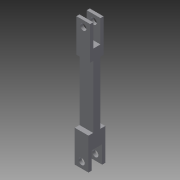
# Autodesk Inventor part: LowerLeg_v2
Saved by Autodesk Inventor 2013 (Build 170138000, 138)
## iProperties
Created: 2012-11-28
Part Number: LowerLeg_v2
Material: Generic
Document SubType Name: Modeling
Designer: Joe
Density: 1 g/cm^3
Author: Joe
Autodesk Inventor part; units mm, degrees
ref_plane "YZ Plane" through (0, 0, 0) normal (1, 0, 0) x (0, 1, 0)
ref_plane "XZ Plane" through (0, 0, 0) normal (0, 1, 0) x (-1, 0, 0)
ref_plane "XY Plane" through (0, 0, 0) normal (0, 0, 1) x (1, 0, 0)
sketch "Sketch1" plane through (0, 0, 0) normal (1, 0, 0) x (0, 1, 0)
  circle A0 centre (0, 0) radius 10
  circle A1 centre (-380, 0) radius 10
  line L0 (0, 0) -> (-380, 0) construction
  line L1 (20, 22.5) -> (-400, 22.5)
  line L2 (-400, 22.5) -> (-400, -22.5)
  line L3 (-400, -22.5) -> (20, -22.5)
  line L4 (20, -22.5) -> (20, 22.5)
  line L5 (20, 0) -> (-400, 0) construction
  dimension "d0" = 380
  dimension "d2" = 20
  dimension "d3" = 20
  dimension "d4" = 20
  dimension "d5" = 20
  dimension "d6" = 45
  constraints: 12 end point, 2 centre point, 2 horizontal, 2 midpoint, 2 parallel, 1 coincident, 1 collinear, 1 perpendicular
  measures "d0" distance of L0.start L0.end
  measures "d2" distance from line of L4 L0.start
  measures "d3" distance from line of L2 L0.end
  measures "d4" diameter of A0
  measures "d5" diameter of A1
  measures "d6" distance of L3.end L1.start
extrude "Extrusion1" add sketch "Sketch1" along normal mid plane 24
sketch "Sketch2" plane through (12, 0, 0) normal (1, 0, 0) x (0, 0, -1)
  circle A0 centre (0, 0) radius 10 projected
  line L0 (22.5, -400) -> (22.5, 20) projected
  line L1 (22.5, 20) -> (-22.5, 20) projected
  line L2 (-22.5, 20) -> (22.5, 20)
  line L3 (22.5, 20) -> (22.5, -90)
  line L4 (22.5, -90) -> (-22.5, -90)
  line L5 (-22.5, -90) -> (-22.5, 20)
  circle A1 centre (0, 0) radius 10
  dimension "d9" = 110
  constraints: 8 end point, 2 parallel, 1 centre point, 1 coincident, 1 concentric, 1 horizontal, 1 perpendicular, 1 point on line
  measures "d9" distance of L4.end L1.end
extrude "Extrusion2" add sketch "Sketch2" along normal blind 10
mirror "Mirror1" about plane through (0, 0, 0) normal (1, 0, 0) of "Extrusion2"
sketch "Sketch3" plane through (-12, -400, 22.5) normal (0, 0, 1) x (1, 0, 0)
  line L0 (34, 420) -> (-10, 420) projected
  line L1 (0, 420) -> (24, 420)
  line L2 (24, 420) -> (24, 345)
  line L3 (24, 345) -> (0, 345)
  line L4 (0, 345) -> (0, 420)
  line L5 (12, 420) -> (12, 345) construction
  point P0 (12, 400)
  dimension "d12" = 24
  dimension "d14" = 75
  constraints: 10 end point, 2 midpoint, 2 parallel, 2 point on line, 1 horizontal, 1 perpendicular
  measures "d12" distance of L2.end L3.end
  measures "d14" distance of L3.end L1.start
extrude "Extrusion3" cut sketch "Sketch3" against normal through all
sketch "Sketch4" plane through (12, 0, 0) normal (1, 0, 0) x (0, 0, -1)
  line L0 (22.5, -400) -> (22.5, -90) projected
  circle A0 centre (0, -380) radius 10 projected
  line L1 (-22.5, -400) -> (22.5, -400)
  line L2 (22.5, -400) -> (22.5, -295)
  line L3 (22.5, -295) -> (-22.5, -295)
  line L4 (-22.5, -295) -> (-22.5, -400)
  circle A1 centre (0, -380) radius 10
  point P0 (0, 0)
  dimension "d18" = 85
  constraints: 8 end point, 2 parallel, 1 centre point, 1 coincident, 1 concentric, 1 horizontal, 1 perpendicular, 1 point on line
  measures "d18" distance from line of A0.centre L3
extrude "Extrusion4" add sketch "Sketch4" along normal blind 15.5
mirror "Mirror2" about plane through (0, 0, 0) normal (1, 0, 0) of "Extrusion4"
sketch "Sketch5" plane through (22, -90, 22.5) normal (0, 0, 1) x (1, 0, 0)
  line L0 (-49.5, -310) -> (5.5, -310) projected
  line L1 (-39.5, -310) -> (-4.5, -310)
  line L2 (-4.5, -310) -> (-4.5, -252)
  line L3 (-4.5, -252) -> (-39.5, -252)
  line L4 (-39.5, -252) -> (-39.5, -310)
  line L5 (-22, -252) -> (-22, -310) construction
  point P0 (-22, 90)
  point P1 (-22, -310)
  dimension "d21" = 35
  dimension "d23" = 58
  constraints: 10 end point, 3 midpoint, 2 parallel, 2 point on line, 1 horizontal, 1 perpendicular
  measures "d21" distance of L2.end L3.end
  measures "d23" distance of L3.end L1.start
extrude "Extrusion5" cut sketch "Sketch5" against normal through all
move or copy body "Move Body1" bodies to move or copy 1 copy no rotation origin (0, 0, 0) rotation axis (1, 0, 0) rotation angle 90
move or copy body "Move Body2" bodies to move or copy 1 copy no rotation origin (0, 0, 0) rotation axis (0, 0, 1) rotation angle 90
body "Solid1"
